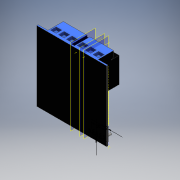
# Autodesk Inventor part: H Bridge #2
Saved by Autodesk Inventor 2016 (Build 200138000, 138)
## iProperties
Created: 2016-05-08
Part Number: H Bridge #2
Material: Generic
Document SubType Name: Modeling
Designer: Kenneth Daniel
Density: 1 g/cm^3
Appearance: Default
Author: Kenneth Daniel
Autodesk Inventor part; units mm, degrees
ref_plane "YZ Plane" through (0, 0, 0) normal (1, 0, 0) x (0, 1, 0)
ref_plane "XZ Plane" through (0, 0, 0) normal (0, 1, 0) x (-1, 0, 0)
ref_plane "XY Plane" through (0, 0, 0) normal (0, 0, 1) x (1, 0, 0)
sketch "Sketch1" plane through (0, 0, 0) normal (0, 1, 0) x (-1, 0, 0)
  line L0 (-25, 25) -> (-25, -25)
  line L1 (-25, -25) -> (25, -25)
  line L2 (25, -25) -> (25, 25)
  line L3 (25, 25) -> (-25, 25)
  line L4 (-25, 25) -> (25, -25) construction
  line L5 (-25, -25) -> (25, 25) construction
  point P0 (0, 0)
  dimension "d0" = 50
  dimension "d1" = 50
  constraints: 12 end point, 2 midpoint, 2 parallel, 1 perpendicular, 1 vertical
  measures "d0" distance of L0.start L0.end
  measures "d1" distance of L1.end L0.end
extrude "Extrusion1" add sketch "Sketch1" along normal blind 1
sketch "Sketch2" plane through (0, 1, 0) normal (0, 1, 0) x (1, 0, 0)
  line L0 (25, -25) -> (25, 25) construction
  line L1 (25, -25) -> (25, -20) construction
  line L2 (25, -20) -> (-25, -20) construction
  line L3 (-25, 25) -> (-25, -25) construction
  line L4 (25, -20) -> (25, -2) construction
  line L5 (25, -2) -> (-25, -2) construction
  line L6 (25, -20) -> (18, -20) construction
  line L7 (18, -20) -> (18, -2) construction
  line L8 (-25, -20) -> (-18, -20) construction
  line L9 (-18, -20) -> (-18, -2) construction
  line L10 (1, -2) -> (-1, -2) construction
  line L11 (-1, -2) -> (-1, -20) construction
  line L12 (-1, -20) -> (1, -20) construction
  line L13 (1, -20) -> (1, -2) construction
  line L14 (1, -2) -> (-1, -20) construction
  line L15 (-1, -2) -> (1, -20) construction
  line L16 (18, -2) -> (1, -2)
  line L17 (1, -2) -> (1, -20)
  line L18 (1, -20) -> (18, -20)
  line L19 (18, -20) -> (18, -2)
  line L20 (-1, -2) -> (-18, -2)
  line L21 (-18, -2) -> (-18, -20)
  line L22 (-18, -20) -> (-1, -20)
  line L23 (-1, -20) -> (-1, -2)
  point P0 (0, 0)
  point P1 (0, -11)
  dimension "d4" = 5
  dimension "d5" = 18
  dimension "d6" = 7
  dimension "d7" = 7
  dimension "d8" = 2
  constraints: 44 end point, 8 point on line, 7 perpendicular, 6 parallel, 3 horizontal, 2 midpoint
  measures "d4" distance of L0.start L1.end
  measures "d5" distance of L1.end L4.end
  measures "d6" distance of L1.end L6.end
  measures "d7" distance of L2.end L8.end
  measures "d8" distance of L10.start L10.end
extrude "Extrusion2" add sketch "Sketch2" along normal blind 15
sketch "Sketch3" plane through (0, 1, 0) normal (0, 1, 0) x (1, 0, 0)
  line L0 (18, -20) -> (1, -20) projected
  line L1 (18, -20) -> (18, -25)
  line L2 (-25, -25) -> (25, -25) projected
  line L3 (1, -20) -> (1, -25)
  line L4 (1, -25) -> (18, -25)
  line L5 (18, -20) -> (1, -20)
  line L6 (18, -25) -> (12.33, -25)
  line L7 (12.33, -25) -> (12.33, -20)
  line L8 (18, -20) -> (12.33, -20)
  line L9 (12.33, -20) -> (6.66, -20)
  line L10 (6.66, -20) -> (6.66, -25)
  line L11 (6.66, -20) -> (1, -20)
  point P0 (0, 0)
  dimension "d11" = 5.67
  dimension "d12" = 5.67
  constraints: 20 end point, 6 point on line, 3 collinear, 3 perpendicular, 1 parallel, 1 vertical
  measures "d11" distance of L1.end L6.end
  measures "d12" distance of L7.end L9.end
extrude "Extrusion3" add sketch "Sketch3" along normal blind 11
sketch "Sketch4" plane through (18, 1, 25) normal (1, 0, 0) x (0, 0, -1)
  line L0 (5, 11) -> (5, 15) projected
  line L1 (5, 11) -> (4, 11)
  line L2 (0, 11) -> (5, 11) projected
  line L3 (4, 11) -> (5, 9.2085)
  line L4 (5, 0) -> (5, 15) projected
  point P0 (25, -1)
  dimension "d9" = 15
  dimension "d15" = 1
  constraints: 4 end point, 2 point on line
  measures "d15" distance of L0.start L1.end
extrude "Extrusion4" cut sketch "Sketch4" against normal through all
sketch "Sketch5" plane through (0, 12, 0) normal (0, 1, 0) x (1, 0, 0)
  line L0 (18, -25) -> (18, -21) construction
  line L1 (18, -21) -> (12.33, -21) construction
  line L2 (18, -21) -> (1, -21) construction
  line L3 (12.33, -21) -> (12.33, -25.0141) construction
  line L4 (12.33, -25.0141) -> (6.66, -25) construction
  line L5 (1, -25) -> (18, -25) construction
  line L6 (6.66, -25) -> (6.67, -21) construction
  line L7 (6.67, -21) -> (1, -21) construction
  line L8 (-25, -25) -> (1, -25) construction
  line L9 (1, -21) -> (1, -25) construction
  circle A0 centre (3.835, -23) radius 1.625
  circle A1 centre (9.5, -23) radius 1.625
  circle A2 centre (15.165, -23) radius 1.625
  point P0 (0, 0)
  dimension "d18" = 5.67
  dimension "d19" = 5.67
  dimension "d20" = 5.67
  dimension "d21" = 3.25
  dimension "d22" = 3.25
  dimension "d23" = 3.25
  constraints: 12 end point, 4 point on line, 3 centre point, 3 perpendicular
  measures "d18" distance of L0.end L1.end
  measures "d19" distance of L3.end L4.end
  measures "d20" distance of L6.end L7.end
  measures "d21" diameter of A0
  measures "d22" diameter of A1
  measures "d23" diameter of A2
extrude "Extrusion5" cut sketch "Sketch5" against normal blind 1.5
sketch "Sketch6" plane through (-25, 0, 25) normal (0, 0, 1) x (1, 0, 0)
  line L0 (0, 1) -> (26, 1) projected
  line L1 (26, 1) -> (43.0101, 1)
  line L2 (26, 12) -> (43, 12) construction
  line L3 (26, 12) -> (31.67, 12) construction
  line L4 (31.67, 12) -> (31.67, 1) construction
  line L5 (31.67, 1) -> (37.34, 1) construction
  line L6 (50, 1) -> (0, 1) construction
  line L7 (37.34, 1) -> (37.34, 12) construction
  line L8 (26.835, 6.1045) -> (30.835, 6.1045)
  line L9 (30.835, 6.1045) -> (30.835, 2.1045)
  line L10 (30.835, 2.1045) -> (26.835, 2.1045)
  line L11 (26.835, 2.1045) -> (26.835, 6.1045)
  line L12 (26.835, 6.1045) -> (30.835, 2.1045) construction
  line L13 (30.835, 6.1045) -> (26.835, 2.1045) construction
  point P0 (25, 0)
  point P1 (28.835, 4.1045)
  dimension "d26" = 5.67
  dimension "d27" = 5.67
  dimension "d28" = 4
  dimension "d29" = 4
  constraints: 22 end point, 4 point on line, 3 perpendicular, 2 horizontal, 2 midpoint, 2 parallel
  measures "d26" distance of L2.start L3.end
  measures "d27" distance of L4.end L5.end
  measures "d28" distance of L8.start L8.end
  measures "d29" distance of L8.end L9.end
extrude "Extrusion6" cut sketch "Sketch6" against normal blind 2
ref_plane "Work Plane1" through (9.5, 1, 2) normal (-1, 0, 0) x (0, 0, 1)
mirror "Mirror1" about plane through (9.5, 1, 2) normal (-1, 0, 0) of "Extrusion6"
ref_plane "Work Plane2" through (6.6675, 1, 2) normal (-1, 0, 0) x (0, 0, 1)
mirror "Mirror2" about plane through (6.6675, 1, 2) normal (-1, 0, 0) of "Extrusion6"
ref_plane "Work Plane3" through (0, 0, -25) normal (-1, 0, 0) x (0, 0, 1)
mirror "Mirror3" about plane through (0, 0, -25) normal (-1, 0, 0) of "Extrusion3", "Extrusion5", "Extrusion6", "Mirror1", "Mirror2", "Extrusion2"
sketch "Sketch7" plane through (0, 1, 0) normal (0, 1, 0) x (1, 0, 0)
  line L0 (25, 25) -> (25, 23) construction
  line L1 (25, -25) -> (25, 25) construction
  line L2 (25, 23) -> (23, 23) construction
  line L3 (23, 23) -> (13, 23)
  line L4 (13, 23) -> (13, 20.4297)
  line L5 (13, 20.4297) -> (23, 20.4297)
  line L6 (23, 20.4297) -> (23, 23)
  line L7 (18, 20.4297) -> (18, 23)
  line L8 (18, 20.4297) -> (23, 20.4297)
  line L9 (20.5, 20.4297) -> (20.5, 23)
  line L10 (18, 20.4297) -> (13, 20.4297)
  line L11 (15.5, 20.4297) -> (15.5, 23)
  circle A0 centre (21.75, 21.6797) radius 1.25
  circle A1 centre (19.25, 21.6797) radius 1.25
  circle A2 centre (16.75, 21.6797) radius 1.25
  circle A3 centre (14.25, 21.6797) radius 1.25
  circle A4 centre (21.75, 21.6797) radius 0.75
  circle A5 centre (19.25, 21.6797) radius 0.75
  circle A6 centre (16.75, 21.6797) radius 0.75
  circle A7 centre (14.25, 21.6797) radius 0.75
  point P0 (0, 0)
  dimension "d33" = 2
  dimension "d34" = 2
  dimension "d35" = 10
  dimension "d36" = 0.5
  dimension "d37" = 0.5
  dimension "d38" = 0.5
  dimension "d39" = 0.5
  constraints: 22 end point, 12 tangent, 8 centre point, 4 midpoint, 4 perpendicular, 3 point on line, 2 collinear, 2 parallel, 1 horizontal
  measures "d33" distance of L0.start L0.end
  measures "d34" distance of L0.end L2.end
  measures "d35" distance of L5.end L4.end
  measures "d36" radial gap between concentric circles of A0 A4
  measures "d37" radial gap between concentric circles of A1 A5
  measures "d38" radial gap between concentric circles of A2 A6
  measures "d39" radial gap between concentric circles of A3 A7
extrude "Extrusion7" add sketch "Sketch7" along normal blind 5 contours A4 | A5 | A6 | A7
extrude "Extrusion8" add sketch "Sketch7" along normal blind 1 contours L6 A0 L9 L3 | L9 A1 L7 L3 | A0 | L6 L5 A0 | L7 A2 L11 L3 | A0 L5 L9 | A1 | L9 L5 A1 | L11 A3 L4 L3 | A1 L5 L7 | A2 | L7 L5 A2 | A2 L5 L11 | A3 | L11 L5 A3 | A3 L5 L4 | A4 | A5 | A6 | A7
body "Solid1"
